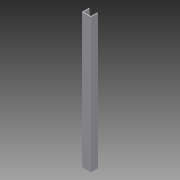
# Autodesk Inventor part: 19in c-channel
Saved by Autodesk Inventor 2013 (Build 170138000, 138)
## iProperties
Created: 2013-01-08
Part Number: 19in c-channel
Material: Generic
Document SubType Name: Modeling
Designer: Naphat
Density: 1 g/cm^3
Author: Naphat
Autodesk Inventor part; units mm, degrees
ref_plane "YZ Plane" through (0, 0, 0) normal (1, 0, 0) x (0, 1, 0)
ref_plane "XZ Plane" through (0, 0, 0) normal (0, 1, 0) x (-1, 0, 0)
ref_plane "XY Plane" through (0, 0, 0) normal (0, 0, 1) x (1, 0, 0)
sketch "Sketch1" plane through (0, 0, 0) normal (0, 0, 1) x (1, 0, 0)
  line L0 (-16, 12.5) -> (-13, 12.5)
  line L1 (-13, 12.5) -> (-13, -9.5)
  line L2 (-13, -9.5) -> (13, -9.5)
  line L3 (13, -9.5) -> (13, 12.9)
  line L4 (13, 12.9) -> (16, 12.9)
  line L5 (16, 12.9) -> (16, -12.5)
  line L6 (16, -12.5) -> (-16, -12.5)
  line L7 (-16, -12.5) -> (-16, 12.5)
  point P0 (0, 0)
  dimension "d0" = 3
  dimension "d2" = 3
  dimension "d3" = 25
  dimension "d4" = 32
  dimension "d5" = 16
  dimension "d7" = 12.5
  dimension "d8" = 3
  constraints: 16 end point, 6 parallel, 1 horizontal, 1 perpendicular
  measures "d0" distance of L0.start L0.end
  measures "d2" distance of L3.end L4.end
  measures "d3" distance of L6.end L0.start
  measures "d4" distance of L5.end L6.end
  measures "d5" distance from line of point (0, 0) L7
  measures "d7" distance from line of L6 point (0, 0)
  measures "d8" distance between parallel lines of L6 L2
extrude "Extrusion1" add sketch "Sketch1" against normal blind 481.1268
sketch "Sketch4" plane through (-16, -12.5, 0) normal (0, -1, 0) x (1, 0, 0)
  line L0 (32, 0) -> (0, 0) projected
  line L1 (32, -481.1268) -> (0, -481.1268) projected
  line L2 (32, 0) -> (32, -481.1268) projected
  circle A0 centre (16, -12.5) radius 3.175
  circle A1 centre (16, -468.6268) radius 3.175
  point P0 (16, 0)
  dimension "d21" = 6.35
  dimension "d22" = 6.35
  dimension "d23" = 12.5
  dimension "d24" = 12.5
  dimension "d25" = 16
  constraints: 2 centre point, 1 vertical alignment
  measures "d21" diameter of A0
  measures "d22" diameter of A1
  measures "d23" distance from line of A0.centre L0
  measures "d24" distance from line of A1.centre L1
  measures "d25" distance from line of L2 A0.centre
hole "Hole1" at (0, -12.5, -12.5) at (0, -12.5, -468.6268) direction (0, 1, 0) diameter 6.35 depth 3 tip angle 118
equation "\"d2\" = d0"
equation "\"d5\" = 0.5 * d4"
equation "\"d7\" = 0.5 * d3"
equation "\"d8\" = d0"
equation "\"d24\" = d23"
body "Solid1"
